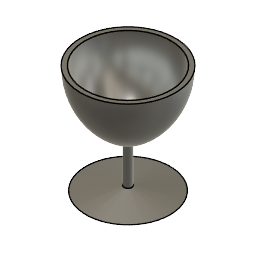
09- CUT SECTION OF SOLIDS_ (Autodesk Fusion 360 design; units mm, degrees)
part number: 2025-12-11-12-31-38-248
Autodesk Fusion 360 part; units mm, degrees
sketch "Sketch1" plane through (0, 0, 0) normal (0, 0, 1) x (1, 0, 0)
  line L0 (0, 0) -> (-1.366, 0)
  line L1 (0, 0) -> (0, 1.501)
  line L2 (-0.123, 1.3896) -> (-0.123, 0.148)
  line L3 (-1.366, 0) -> (-0.123, 0.148)
  line L4 (-1.5393, 3.52) -> (-1.3912, 3.52)
  arc A0 (-1.3912, 3.52) -> (0, 1.501) centre (0.7215, 3.487) ccw
  arc A1 (-1.5393, 3.52) -> (-0.123, 1.3896) centre (0.7215, 3.487) ccw
  point P0 (0.7215, 3.487)
  dimension "d1" = 1.366
  dimension "d2" = 1.501
  dimension "d4" = 1.986
  dimension "d5" = 4.226
  dimension "d6" = 4.522
  dimension "d7" = 0.123
  dimension "d8" = 0.148
  constraint coincident L0.start L1.start
  constraint horizontal L0
  constraint perpendicular L0 L1
  constraint coincident P0 A0.centre
  constraint perpendicular L0 L2
  measures "d1" distance of L0.start L0.end
  measures "d2" distance of L0.start L1.end
  measures "d4" vertical distance of L1.end P0
  measures "d5" diameter of A0
  measures "d6" diameter of A1
  measures "d7" distance of L1 L2
  measures "d8" distance of L0 L2.end
revolve "Revolve1" add sketch "Sketch1" angle 360 about axis through (0, 0, 0) along (0, 1, 0)
